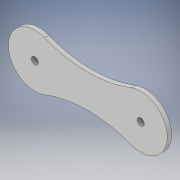
# Autodesk Inventor part: pierna1
Saved by Autodesk Inventor 2019 (Build 230136000, 136)
## iProperties
Created: 2020-02-11
Part Number: pierna1
Material: Generic
Document SubType Name: Modeling
Designer: jacqu
Density: 1 g/cm^3
Appearance: Default
radio_muslo: 20.000 mm
curva: 90.000 mm
distancia_centros: 80.000 mm
espesor: 3.300 mm
Author: jacqu
Autodesk Inventor part; units mm, degrees
ref_plane "YZ Plane" through (0, 0, 0) normal (1, 0, 0) x (0, 1, 0)
ref_plane "XZ Plane" through (0, 0, 0) normal (0, 1, 0) x (-1, 0, 0)
ref_plane "XY Plane" through (0, 0, 0) normal (0, 0, 1) x (1, 0, 0)
sketch "Sketch1" plane through (0, 0, 0) normal (0, 0, 1) x (1, 0, 0)
  arc A0 (7.2727, 18.6308) -> (7.2727, -18.6308) centre (0, 0) ccw
  arc A1 (7.2727, 18.6308) -> (72.7273, 18.6308) centre (40, 102.4695) ccw
  arc A2 (72.7273, -18.6308) -> (7.2727, -18.6308) centre (40, -102.4695) ccw
  arc A3 (72.7273, -18.6308) -> (72.7273, 18.6308) centre (80, 0) ccw
  circle A4 centre (0, 0) radius 2.65
  circle A5 centre (80, 0) radius 2.65
  dimension "radio_muslo" = 20
  dimension "curva" = 90
  dimension "d2" = 90
  dimension "d3" = 20
  dimension "d4" = 5.3
  dimension "d5" = 5.3
  dimension "distancia_centros" = 80
  constraints: 8 point on circle, 6 centre point, 4 tangent, 2 concentric, 1 coincident, 1 horizontal alignment
  measures "radio_muslo" radius of A0
  measures "curva" radius of A1
  measures "d2" radius of A2
  measures "d3" radius of A3
  measures "d4" diameter of A4
  measures "d5" diameter of A5
  measures "distancia_centros" distance of A3.centre point (0, 0)
extrude "Extrusion1" add sketch "Sketch1" along normal blind 3.3
equation "\"d2\" = curva"
equation "\"d3\" = radio_muslo"
equation "\"d5\" = d4"
body "Solid1"
